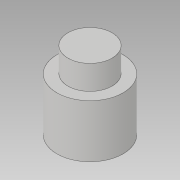
# Autodesk Inventor part: locking_spud
Saved by Autodesk Inventor 2019.3 (Build 233278000, 278)
## iProperties
Created: 2019-03-03
Part Number: locking_spud
Material: Generic
Document SubType Name: Modeling
Designer: WW
Density: 1 g/cm^3
Appearance: Default
Author: WW
Autodesk Inventor part; units mm, degrees
ref_plane "YZ Plane" through (0, 0, 0) normal (1, 0, 0) x (0, 1, 0)
ref_plane "XZ Plane" through (0, 0, 0) normal (0, 1, 0) x (-1, 0, 0)
ref_plane "XY Plane" through (0, 0, 0) normal (0, 0, 1) x (1, 0, 0)
sketch "Sketch1" plane through (0, 0, 0) normal (0, 0, 1) x (1, 0, 0)
  line L0 (0, 0) -> (0, -23.3581)
  line L1 (0, 0) -> (3.75, 0)
  line L2 (3.75, 0) -> (3.75, 6)
  line L3 (3.75, 6) -> (0, 6)
  line L4 (0, 6) -> (0, 0)
  line L5 (0, 6) -> (0, 6.0616)
  arc A0 (3.75, 6) -> (0, 6.0616) centre (0, -108.1884) ccw
  line L6 (2.5, 6.0342) -> (2.5, 8.7848)
  line L7 (2.5, 8.7848) -> (0, 8.7848)
  arc A1 (2.5, 8.7848) -> (0, 8.8116) centre (0, -108.1884) ccw
  line L8 (0, 8.8116) -> (0, 8.7848)
  line L9 (0, 8.7848) -> (0, 6.0616)
  dimension "d0" = 5
  dimension "d1" = 114.25
  dimension "d2" = 7.5
  dimension "d3" = 6
  dimension "d4" = 117
  constraints: 20 end point, 5 point on circle, 4 vertical, 3 perpendicular, 2 centre point, 2 line through centre, 1 collinear, 1 concentric, 1 horizontal, 1 point on line
  measures "d0" diameter of L6 L0
  measures "d1" radius of A0
  measures "d2" diameter of L2 L0
  measures "d3" distance between parallel lines of L1 L3
  measures "d4" radius of A1
revolve "Revolution1" add sketch "Sketch1" angle 360 about axis through (0, 0, 0) along (0, -1, 0)
body "Solid1"
